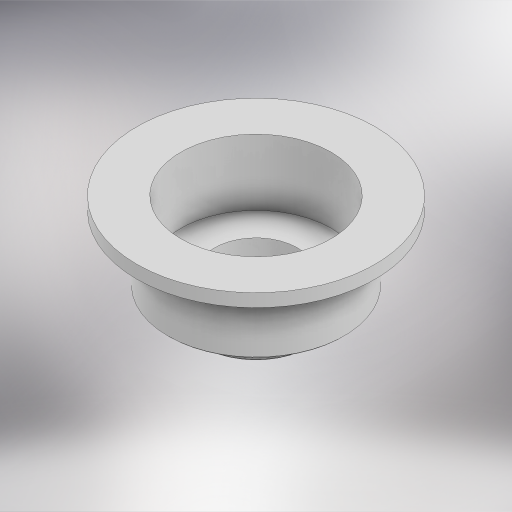
# Autodesk Inventor part: Topf
Saved by Autodesk Inventor 2023 (Build 270158000, 158)
## iProperties
Created: 2022-12-28
Part Number: Topf
Material: Generisch
Document SubType Name: Modeling
Designer: schil
Density: 1 g/cm^3
Appearance: Vorgabe
Author: schil
Autodesk Inventor part; units mm, degrees
ref_plane "YZ Plane" through (0, 0, 0) normal (1, 0, 0) x (0, 1, 0)
ref_plane "XZ Plane" through (0, 0, 0) normal (0, 1, 0) x (-1, 0, 0)
ref_plane "XY Plane" through (0, 0, 0) normal (0, 0, 1) x (1, 0, 0)
sketch "Skizze1" plane through (0, 0, 0) normal (1, 0, 0) x (0, 1, 0)
  line L0 (0, -16) -> (-5, -16)
  line L1 (-5, -16) -> (-5, -34)
  line L2 (-5, -34) -> (0, -34)
  line L3 (0, -34) -> (0, -16)
  line L4 (-11.0954, 0) -> (31.5723, 0) projected
  line L5 (0, -55.2) -> (0, 9.2) projected
  line L6 (0, -34) -> (25.477, -34)
  line L7 (25.477, -34) -> (25.477, -29)
  line L8 (25.477, -29) -> (0, -29)
  line L9 (0, -29) -> (0, -34)
  line L10 (25.477, -34) -> (20.477, -34)
  line L11 (20.477, -34) -> (20.477, -46)
  line L12 (20.477, -46) -> (25.477, -46)
  line L13 (25.477, -46) -> (25.477, -34)
  point P0 (0, 0)
  point P1 (0, -29)
  dimension "d0" = 16
  dimension "d1" = 34
  dimension "d2" = 5
  dimension "d3" = 5
  dimension "d4" = 5
  dimension "d5" = 46
  constraints: 24 end point, 6 parallel, 3 horizontal, 3 perpendicular, 1 point on line
  measures "d0" distance between parallel lines of L4 L0
  measures "d1" distance between parallel lines of L2 L4
  measures "d2" distance between parallel lines of L1 L3
  measures "d3" distance between parallel lines of L6 L8
  measures "d4" distance between parallel lines of L11 L13
  measures "d5" distance between parallel lines of L12 L4
revolve "Umdrehung1" add sketch "Skizze1" angle 360 about axis through (0, -10, 0) along (0, 1, 0)
chamfer "Fase1" distance 0.5 angle 45 1 edges at (0, -5, 34)
sketch "Skizze2" plane through (0, -5, 0) normal (0, -1, 0) x (1, 0, 0)
  circle A0 centre (0, 0) radius 16
  circle A1 centre (0, 0) radius 21
  circle A2 centre (0, 0) radius 16 projected
  dimension "d10" = 5
  dimension "d11" = 0
  constraints: 2 centre point, 2 coincident
  measures "d10" radial gap between concentric circles of A0 A1
  measures "d11" radial gap between concentric circles of A2 A0
extrude "Extrusion1" add sketch "Skizze2" along normal blind 10
chamfer "Fase2" distance 0.5 angle 45 2 edges at (-21, -15, 0) (-16, -15, 0)
equation "\"d3\" = d2"
equation "\"d4\" = d2"
